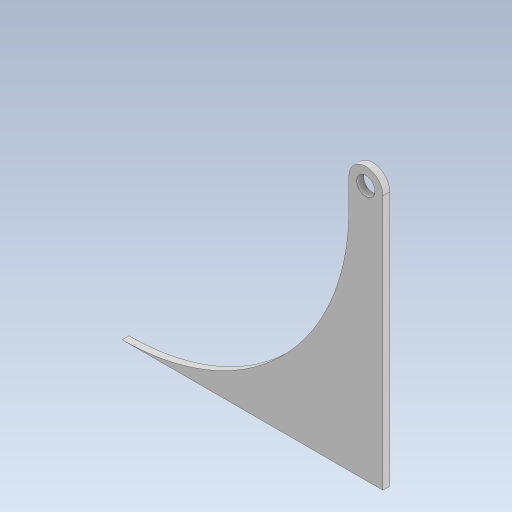
# Autodesk Inventor part: 零件10
Saved by Autodesk Inventor 2023 (Build 270158000, 158)
## iProperties
Created: 2023-05-16
Part Number: 零件10
Material: 一般
Document SubType Name: Modeling
Designer: Johnny Jou
Density: 1 g/cm^3
Appearance: 預設
Author: Johnny Jou
Autodesk Inventor part; units mm, degrees
ref_plane "YZ Plane" through (0, 0, 0) normal (1, 0, 0) x (0, 1, 0)
ref_plane "XZ Plane" through (0, 0, 0) normal (0, 1, 0) x (-1, 0, 0)
ref_plane "XY Plane" through (0, 0, 0) normal (0, 0, 1) x (1, 0, 0)
sketch "草圖1" plane through (0, 0, 0) normal (0, 0, 1) x (1, 0, 0)
  line L0 (0, -80) -> (100, -80)
  arc A0 (100, -80) -> (200, 20) centre (100, 20) ccw
  line L1 (200, 20) -> (200, 40)
  line L2 (200, 40) -> (100, 40)
  line L3 (100, 40) -> (100, -80)
  line L4 (100, -80) -> (200, -80)
  line L5 (200, -80) -> (200, 40)
  line L6 (200, 40) -> (215, 40)
  line L7 (215, 40) -> (215, -80)
  line L8 (215, -80) -> (200, -80)
  line L9 (200, -80) -> (200, 40)
  circle A1 centre (207.5, 32.5) radius 7.5
  circle A2 centre (207.5, 32.5) radius 4
  point P0 (215, 32.5)
  point P1 (200, 32.5)
  dimension "d0" = 8
  dimension "d1" = 15
  constraints: 20 end point, 4 parallel, 3 centre point, 3 horizontal, 3 tangent, 2 perpendicular, 2 point on circle, 1 coincident, 1 collinear, 1 vertical, 5 other
  measures "d0" diameter of A2
  measures "d1" diameter of A1
extrude "擠出1" add sketch "草圖1" along normal blind 3 contours A0 L5 L4 | L1 A1 L7 L8 L5 | A1
